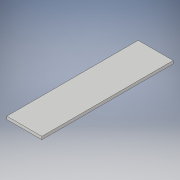
# Autodesk Inventor part: Predni_strana
Saved by Autodesk Inventor 2019 (Build 230136000, 136)
## iProperties
Created: 2021-01-08
Part Number: Predni_strana
Material: Všeobecné
Document SubType Name: Modeling
Designer: Pokor
Density: 1 g/cm^3
Appearance: Výchozí
Author: Pokor
Autodesk Inventor part; units mm, degrees
ref_plane "YZ Plane" through (0, 0, 0) normal (1, 0, 0) x (0, 1, 0)
ref_plane "XZ Plane" through (0, 0, 0) normal (0, 1, 0) x (-1, 0, 0)
ref_plane "XY Plane" through (0, 0, 0) normal (0, 0, 1) x (1, 0, 0)
sketch "Náčrt1" plane through (0, 0, 0) normal (0, 1, 0) x (-1, 0, 0)
  line L0 (0, 0) -> (120, 0)
  line L1 (120, 0) -> (120, -450)
  line L2 (120, -450) -> (0, -450)
  line L3 (0, -450) -> (0, 0)
  dimension "d0" = 120
  dimension "d1" = 450
  constraints: 8 end point, 2 parallel, 1 horizontal, 1 perpendicular
  measures "d0" distance of L1.end L2.end
  measures "d1" distance of L0.end L1.end
extrude "Vysunutí1" add sketch "Náčrt1" along normal blind 10
